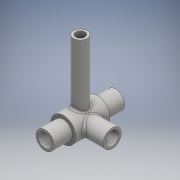
# Autodesk Inventor part: Steam Inlet T Connector
Saved by Autodesk Inventor 2016 (Build 200138000, 138)
## iProperties
Created: 2016-12-04
Part Number: Steam Inlet T Connector
Material: Generic
Document SubType Name: Modeling
Designer: Muhammad
Density: 1 g/cm^3
Appearance: Default
Author: Muhammad
Autodesk Inventor part; units mm, degrees
sketch "Sketch1" plane through (0, 0, 0) normal (0, 1, 0) x (-1, 0, 0)
  circle A0 centre (0, 0) radius 5.5
  dimension "d0" = 11
  constraints: 1 centre point, 1 coincident
  measures "d0" diameter of A0
extrude "Extrusion1" add sketch "Sketch1" along normal blind 15
ref_plane "Work Plane1" through (14, 0, 0) normal (1, 0, 0) x (0, 1, 0)
sketch "Sketch2" plane through (14, 0, 0) normal (1, 0, 0) x (0, 1, 0)
  line L0 (0, 0) -> (7.5, 0)
  circle A0 centre (7.5, 0) radius 3
  circle A1 centre (7.5, 0) radius 4
  dimension "d4" = 7.5
  dimension "d5" = 6
  dimension "d6" = 8
  constraints: 2 centre point, 2 coincident, 2 end point, 1 horizontal
  measures "d4" distance of L0.start L0.end
  measures "d5" diameter of A0
  measures "d6" diameter of A1
extrude "Extrusion2" add sketch "Sketch2" against normal up to surface
ref_plane "Work Plane2" through (0, 7.5, 0) normal (0, 1, 0) x (-1, 0, 0)
sketch "Sketch3" plane through (0, 7.5, 0) normal (0, 1, 0) x (-1, 0, 0)
  circle A0 centre (0, 0) radius 4
  dimension "d10" = 8
  constraints: 1 centre point, 1 coincident
  measures "d10" diameter of A0
extrude "Extrusion3" add sketch "Sketch3" along normal mid plane 31
sketch "Sketch4" plane through (0, -8, 0) normal (0, -1, 0) x (1, 0, 0)
  circle A0 centre (0, 0) radius 3
  dimension "d13" = 6
  constraints: 1 centre point, 1 coincident
  measures "d13" diameter of A0
extrude "Extrusion4" cut sketch "Sketch4" against normal through all
ref_plane "Work Plane3" through (0, 0, 32.5) normal (0, 0, 1) x (1, 0, 0)
sketch "Sketch5" plane through (0, 0, 32.5) normal (0, 0, 1) x (1, 0, 0)
  line L0 (5.5, 15) -> (-5.5, 15) projected
  line L1 (0, 15) -> (0, 7.5)
  circle A0 centre (0, 7.5) radius 3
  circle A1 centre (0, 7.5) radius 2
  point P0 (0, 0)
  dimension "d17" = 7.5
  dimension "d18" = 6
  dimension "d19" = 4
  constraints: 2 centre point, 2 coincident, 2 end point, 1 midpoint, 1 vertical
  measures "d17" distance of L1.start L1.end
  measures "d18" diameter of A0
  measures "d19" diameter of A1
extrude "Extrusion5" add sketch "Sketch5" against normal up to surface
fillet "Fillet1" radius 1 2 edges at (-3, 7.504, 4.6098) (5.5, 3.5, 0.015)
body "Solid1"
